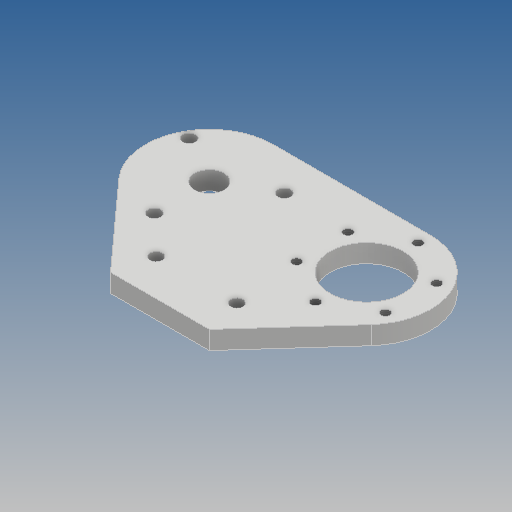
# Autodesk Inventor part: Zylinderplatte
Saved by Autodesk Inventor 2018 (Build 220112000, 112)
## iProperties
Created: 2018-09-25
Part Number: Zylinderplatte
Material: Generisch
Document SubType Name: Modeling
Designer: M.Knabel
Density: 1 g/cm^3
Appearance: Vorgabe
Mass: 13.9598 g
Surface Area: 75.9405 cm^2
Volume: 13.9598 cm^3
Author: M.Knabel
Autodesk Inventor part; units mm, degrees
note: some values were not read from the file. Chosen so that the rebuilt part matches the saved one: direction of "Bohrung1"; direction of "Bohrung2".
ref_plane "YZ Plane" through (0, 0, 0) normal (1, 0, 0) x (0, 1, 0)
ref_plane "XZ Plane" through (0, 0, 0) normal (0, 1, 0) x (-1, 0, 0)
ref_plane "XY Plane" through (0, 0, 0) normal (0, 0, 1) x (1, 0, 0)
sketch "Skizze1" plane through (0, 0, 0) normal (0, 0, 1) x (1, 0, 0)
  line L0 (0, -63.8443) -> (0, 15.5659) projected
  line L1 (-61.5828, 0) -> (61.5828, 0) projected
  line L2 (-13.5, -52.5) -> (13.5, -52.5)
  line L3 (13.5, -52.5) -> (34.4955, -29.2204)
  line L4 (-13.5, -52.5) -> (-34.4955, -29.2204)
  arc A0 (-21.5, 0) -> (-34.4955, -29.2204) centre (-21.5, -17.5) ccw
  arc A1 (34.4955, -29.2204) -> (21.5, 0) centre (21.5, -17.5) ccw
  line L5 (-21.5, 0) -> (21.5, 0)
  point P0 (0, 0)
  dimension "d0" = 43
  dimension "d1" = 27
  dimension "d2" = 35
  dimension "d3" = 17.5
  constraints: 8 end point, 4 point on circle, 4 tangent, 3 point on line, 3 symmetric about line, 2 centre point, 1 collinear, 1 horizontal
  measures "d0" distance of A1.centre A0.centre
  measures "d1" distance of L2.end L2.start
  measures "d2" distance from line of L2 A1.centre
  measures "d3" radius of A0
extrude "Extrusion1" add sketch "Skizze1" along normal blind 5
sketch "Skizze2" plane through (0, 0, 5) normal (0, 0, 1) x (1, 0, 0)
  line L0 (-61.5828, 0) -> (61.5828, 0) projected
  line L1 (0, -63.8443) -> (0, 15.5659) projected
  arc A0 (-21.5, 0) -> (-34.4955, -29.2204) centre (-21.5, -17.5) ccw projected
  circle A1 centre (-21.5, -17.5) radius 4
  arc A2 (34.4955, -29.2204) -> (21.5, 0) centre (21.5, -17.5) ccw projected
  circle A3 centre (21.5, -17.5) radius 10
  circle A4 centre (-11, -42.5) radius 1.7
  circle A5 centre (11, -42.5) radius 1.7
  line L2 (-13.5, -52.5) -> (13.5, -52.5) projected
  point P0 (0, 0)
  dimension "d7" = 8
  dimension "d8" = 20
  dimension "d9" = 3.4
  dimension "d10" = 3.4
  dimension "d11" = 10
  dimension "d12" = 22
  constraints: 4 centre point, 2 coincident, 1 symmetric about line
  measures "d7" diameter of A1
  measures "d8" diameter of A3
  measures "d9" diameter of A4
  measures "d10" diameter of A5
  measures "d11" distance from line of L2 A5.centre
  measures "d12" distance of A5.centre A4.centre
extrude "Extrusion2" cut sketch "Skizze2" against normal up to next
sketch "Skizze3" plane through (0, 0, 5) normal (0, 0, 1) x (1, 0, 0)
  arc A0 (-21.5, 0) -> (-34.4955, -29.2204) centre (-21.5, -17.5) ccw construction
  circle A1 centre (-21.5, -17.5) radius 15 construction
  line L0 (-21.5, -2.5) -> (-21.5, -32.5) construction
  point P0 (0, 0)
  dimension "d15" = 30
  constraints: 2 coincident, 2 end point, 2 point on circle, 1 centre point, 1 midpoint, 1 vertical
  measures "d15" diameter of A1
hole "Bohrung1" at (-21.5, -32.5, 5) direction (0, 0, -1) diameter 3.5 end up to surface
pattern_circular "Runde Anordnung1" count 3 over 360 about axis through (-21.5, -17.5, 5) along (0, 0, -1) of "Bohrung1"
sketch "Skizze4" plane through (0, 0, 5) normal (0, 0, 1) x (1, 0, 0)
  arc A0 (34.4955, -29.2204) -> (21.5, 0) centre (21.5, -17.5) ccw construction
  circle A1 centre (21.5, -17.5) radius 14 construction
  line L0 (21.5, -3.5) -> (21.5, -31.5) construction
  point P0 (0, 0)
  dimension "d26" = 28
  constraints: 2 coincident, 2 end point, 2 point on circle, 1 centre point, 1 midpoint, 1 vertical
  measures "d26" diameter of A1
hole "Bohrung2" at (21.5, -31.5, 5) direction (0, 0, -1) diameter 2.459 end up to surface thread size "M3x0.5" class "6H" standard "ISO Metric profile"
pattern_circular "Runde Anordnung2" count 6 over 360 about axis through (21.5, -17.5, 5) along (0, 0, -1) of "Bohrung2"
